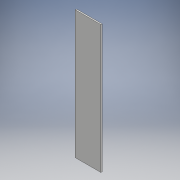
# Autodesk Inventor part: 5050-led-strip
Saved by Autodesk Inventor 2018 (Build 220112000, 112)
## iProperties
Created: 2017-10-10
Part Number: 5050-led-strip
Material: Generic
Document SubType Name: Modeling
Designer: leo2a
Density: 1 g/cm^3
Appearance: Default
Author: leo2a
Autodesk Inventor part; units mm, degrees
ref_plane "YZ Plane" through (0, 0, 0) normal (1, 0, 0) x (0, 1, 0)
ref_plane "XZ Plane" through (0, 0, 0) normal (0, 1, 0) x (-1, 0, 0)
ref_plane "XY Plane" through (0, 0, 0) normal (0, 0, 1) x (1, 0, 0)
sketch "Sketch1" plane through (0, 0, 0) normal (0, 1, 0) x (-1, 0, 0)
  line L0 (-5, 25) -> (-5, -25)
  line L1 (-5, -25) -> (5, -25)
  line L2 (5, -25) -> (5, 25)
  line L3 (5, 25) -> (-5, 25)
  line L4 (-5, 25) -> (5, -25) construction
  line L5 (-5, -25) -> (5, 25) construction
  point P0 (0, 0)
  dimension "d0" = 50
  dimension "d1" = 10
  constraints: 12 end point, 2 midpoint, 2 parallel, 1 perpendicular, 1 vertical
  measures "d0" distance of L0.start L0.end
  measures "d1" distance of L1.end L0.end
extrude "Extrusion1" add sketch "Sketch1" along normal blind 0.5
sketch "Sketch2" plane through (0, 0.5, 0) normal (0, 1, 0) x (1, 0, 0)
  line L0 (2.5, -2.5) -> (2.5, 2.5)
  line L1 (2.5, 2.5) -> (-2.5, 2.5)
  line L2 (-2.5, 2.5) -> (-2.5, -2.5)
  line L3 (-2.5, -2.5) -> (2.5, -2.5)
  line L4 (2.5, -2.5) -> (-2.5, 2.5) construction
  line L5 (2.5, 2.5) -> (-2.5, -2.5) construction
  line L6 (-5, -25) -> (5, -25) projected
  line L7 (0, -25) -> (0, -17)
  line L8 (2.5, -19.5) -> (2.5, -14.5)
  line L9 (2.5, -14.5) -> (-2.5, -14.5)
  line L10 (-2.5, -14.5) -> (-2.5, -19.5)
  line L11 (-2.5, -19.5) -> (2.5, -19.5)
  line L12 (2.5, -19.5) -> (-2.5, -14.5) construction
  line L13 (2.5, -14.5) -> (-2.5, -19.5) construction
  line L14 (5, 25) -> (-5, 25) projected
  line L15 (0, 25) -> (0, 17)
  line L16 (2.5, 14.5) -> (2.5, 19.5)
  line L17 (2.5, 19.5) -> (-2.5, 19.5)
  line L18 (-2.5, 19.5) -> (-2.5, 14.5)
  line L19 (-2.5, 14.5) -> (2.5, 14.5)
  line L20 (2.5, 14.5) -> (-2.5, 19.5) construction
  line L21 (2.5, 19.5) -> (-2.5, 14.5) construction
  point P0 (0, 0)
  dimension "d4" = 5
  dimension "d5" = 5
  dimension "d6" = 8
  dimension "d7" = 5
  dimension "d8" = 5
  dimension "d9" = 8
  dimension "d10" = 5
  constraints: 40 end point, 8 midpoint, 6 parallel, 4 vertical, 3 perpendicular
  measures "d4" distance of L0.start L0.end
  measures "d5" distance of L1.end L0.end
  measures "d6" distance of L7.start L7.end
  measures "d7" distance of L8.start L8.end
  measures "d8" distance of L9.end L8.end
  measures "d9" distance of L15.start L15.end
  measures "d10" distance of L16.start L16.end
extrude "Extrusion2" add sketch "Sketch2" along normal blind 1
sketch "Sketch3" plane through (0, 0.5, 0) normal (0, 1, 0) x (1, 0, 0)
  line L0 (-5, -25) -> (5, -25) projected
  line L1 (0, -25) -> (0, -11)
  line L2 (1.7, -11.65) -> (1.7, -10.35)
  line L3 (1.7, -10.35) -> (-1.7, -10.35)
  line L4 (-1.7, -10.35) -> (-1.7, -11.65)
  line L5 (-1.7, -11.65) -> (1.7, -11.65)
  line L6 (1.7, -11.65) -> (-1.7, -10.35) construction
  line L7 (1.7, -10.35) -> (-1.7, -11.65) construction
  line L8 (0, -11) -> (0, -6)
  line L9 (1.9118, -6.65) -> (-1.9118, -6.65)
  line L10 (-1.9118, -6.65) -> (-1.9118, -5.35)
  line L11 (-1.9118, -5.35) -> (1.9118, -5.35)
  line L12 (1.9118, -5.35) -> (1.9118, -6.65)
  line L13 (1.9118, -6.65) -> (-1.9118, -5.35) construction
  line L14 (-1.9118, -6.65) -> (1.9118, -5.35) construction
  line L15 (2.5, 2.5) -> (-2.5, 2.5) projected
  line L16 (0, 2.5) -> (0, 8.5)
  line L17 (1.9118, 7.85) -> (-1.9118, 7.85)
  line L18 (-1.9118, 7.85) -> (-1.9118, 9.15)
  line L19 (-1.9118, 9.15) -> (1.9118, 9.15)
  line L20 (1.9118, 9.15) -> (1.9118, 7.85)
  line L21 (1.9118, 7.85) -> (-1.9118, 9.15) construction
  line L22 (-1.9118, 7.85) -> (1.9118, 9.15) construction
  point P0 (0, 0)
  dimension "d13" = 14
  dimension "d14" = 1.3
  dimension "d15" = 3.4
  dimension "d16" = 5
  dimension "d17" = 1.3
  dimension "d18" = 6
  dimension "d19" = 1.3
  constraints: 42 end point, 8 midpoint, 6 parallel, 4 vertical, 3 perpendicular, 2 horizontal
  measures "d13" distance of L1.start L1.end
  measures "d14" distance of L2.start L2.end
  measures "d15" distance of L3.end L2.end
  measures "d16" distance of L1.end L8.end
  measures "d17" distance of L9.end L10.end
  measures "d18" distance of L16.start L16.end
  measures "d19" distance of L17.end L18.end
extrude "Extrusion3" add sketch "Sketch3" along normal blind 0.5
sketch "Sketch4" plane through (0, 1.5, 0) normal (0, 1, 0) x (1, 0, 0)
  circle A0 centre (0, 0) radius 2
  circle A1 centre (0, -17) radius 2
  circle A2 centre (0, 17) radius 2
  dimension "d22" = 4
  dimension "d23" = 4
  dimension "d24" = 4
  constraints: 3 centre point, 1 coincident
  measures "d22" diameter of A0
  measures "d23" diameter of A1
  measures "d24" diameter of A2
extrude "Extrusion4" cut sketch "Sketch4" against normal blind 0.1
body "Solid1"
